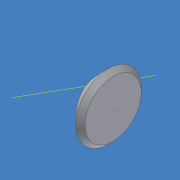
# Autodesk Inventor part: bevelgear_wheel2
Saved by Autodesk Inventor 2011 (Build 150239000, 239)
## iProperties
Created: 2005-03-17
Part Number: bevelgear_wheel2
Document SubType Name: Modeling
Designer: Miroslav Petele
Density: 1 g/cm^3
Control State: 0
Master: False
Checked Out: False
Shininess: 64.0
Angle Display Precision: 2
Document Length Units: 11269
Document Angle Units: 11279
Document Time Units: 11290
Document Mass Units: 11283
Document Length Units Precision: 3
Document Angle Units Precision: 2
Density: 0.0
Volumn: 0.0
Area: 0.0
PropertySet Name: Model Information
Author: Miroslav Petele
Autodesk Inventor part; units mm, degrees
ref_plane "YZ Plane" through (0, 0, 0) normal (1, 0, 0) x (0, 1, 0)
ref_plane "XZ Plane" through (0, 0, 0) normal (0, 1, 0) x (-1, 0, 0)
ref_plane "XY Plane" through (0, 0, 0) normal (0, 0, 1) x (1, 0, 0)
ref_plane "Work Plane1" through (0, 0, -10) normal (-0.8660254, 0.5, 0) x (-0.5, -0.8660254, 0)
sketch "Sketch1" plane through (0, 0, 0) normal (0, 0, 1) x (1, 0, 0)
  line L0 (-8.9539, 0) -> (116.4008, 0) projected
  line L1 (0, 0) -> (22.3574, 21.64) construction
  line L2 (67.2393, 58.2059) -> (103.4352, 89.5391)
  line L3 (67.2393, 58.2059) -> (68.9265, 56.4627)
  line L4 (68.9265, 56.4627) -> (68.9265, 0)
  line L5 (103.4352, 89.5391) -> (109.1987, 83.5845)
  line L6 (109.1987, 83.5845) -> (109.1987, 0)
  dimension "delta" = 44.066
  dimension "hxe" = 8.287
  dimension "hxi" = 2.426
  dimension "hfe" = 7.6
  dimension "hfi" = 4.9405
  dimension "Ri" = 88.7955
  dimension "b" = 47.8
  constraints: 12 end point, 4 perpendicular, 2 point on line
  measures "delta" angle of L0 L1
  measures "hxe" distance of L2.end L5.end
  measures "hxi" distance of L2.start L3.end
  measures "hfe" distance from line of L1 L2.end
  measures "hfi" distance from line of L1 L2.start
  measures "Ri" distance from line of L1.start L3
  measures "b" distance between parallel lines of L5 L3
revolve "Revolution1" add sketch "Sketch1" angle 360 about axis through (-10, 0, 0) along (1, 0, 0)
sketch "Sketch2" plane through (0, 0, 0) normal (0, 0, 1) x (1, 0, 0)
  line L0 (-9.7443, 0) -> (126.676, 0) projected
  line L1 (0, 0) -> (23.1863, 22.4423) construction
  line L2 (67.2393, 58.2059) -> (103.4352, 89.5391) projected
  line L3 (67.2393, 58.2059) -> (62.2661, 63.344)
  line L4 (103.4352, 89.5391) -> (95.7849, 97.443)
  line L5 (95.7849, 97.443) -> (62.2661, 63.344)
  dimension "hae" = 3.4
  dimension "hai" = 2.2102
  dimension "d10" = 44.066
  constraints: 8 end point, 1 parallel, 1 perpendicular
  measures "hae" distance from line of L1 L4.end
  measures "hai" distance from line of L1 L3.end
  measures "d10" angle of L0 L1
revolve "Revolution2" add sketch "Sketch2" angle 360 about axis through (-10, 0, 0) along (1, 0, 0)
equation "\"delta\" = MC_delta2"
equation "\"hxe\" = MC_hxe2 + MC_hae2 - MC_h2E"
equation "\"hxi\" = MC_hxi2 + MC_hai2 - MC_h2A"
equation "\"hfe\" = MC_h2E - MC_hae2"
equation "\"hfi\" = MC_h2A - MC_hai2"
equation "\"Ri\" = MC_Ri"
equation "\"b\" = MC_b"
equation "\"hae\" = MC_hae2"
equation "\"hai\" = MC_hai2"
equation "\"d10\" = delta"
equation "\"SumDelta\" = MC_deltasum"
equation "\"MC_deltasum\" = 60deg"
equation "\"MC_b\" = 47.8"
equation "\"MC_Ri\" = 88.79551"
equation "\"MC_alfa\" = 20deg"
equation "\"MC_delta1\" = 15.934197deg"
equation "\"MC_hae1\" = 6.6"
equation "\"MC_hxe1\" = 9.9"
equation "\"MC_hai1\" = 4.29041"
equation "\"MC_hxi1\" = 4.84827"
equation "\"MC_delta2\" = 44.0658deg"
equation "\"MC_hae2\" = 3.4"
equation "\"MC_hxe2\" = 15.887"
equation "\"MC_hai2\" = 2.21021"
equation "\"MC_hxi2\" = 7.36647"
equation "\"MC_Ang1A\" = 212.432024deg"
equation "\"MC_Ang1B\" = 194.292538deg"
equation "\"MC_Ang1C\" = 180deg"
equation "\"MC_Ang1D\" = 168.447967deg"
equation "\"MC_Ang1E\" = 158.917183deg"
equation "\"MC_Ang2A\" = 167.197885deg"
equation "\"MC_Ang2B\" = 174.358209deg"
equation "\"MC_Ang2C\" = 180deg"
equation "\"MC_Ang2D\" = 184.560013deg"
equation "\"MC_Ang2E\" = 188.322165deg"
equation "\"MC_h1A\" = 7.15068"
equation "\"MC_h1B\" = 8.11301"
equation "\"MC_h1C\" = 9.07534"
equation "\"MC_h1D\" = 10.03767"
equation "\"MC_h1E\" = 11"
equation "\"MC_h2A\" = 7.15068"
equation "\"MC_h2B\" = 8.11301"
equation "\"MC_h2C\" = 9.07534"
equation "\"MC_h2D\" = 10.03767"
equation "\"MC_h2E\" = 11"
equation "\"MC_Rz1A\" = 24.37731"
equation "\"MC_Rz1B\" = 27.65799"
equation "\"MC_Rz1C\" = 30.93866"
equation "\"MC_Rz1D\" = 34.21933"
equation "\"MC_Rz1E\" = 37.5"
equation "\"MC_Rz2A\" = 61.75586"
equation "\"MC_Rz2B\" = 70.0669"
equation "\"MC_Rz2C\" = 78.37793"
equation "\"MC_Rz2D\" = 86.68897"
equation "\"MC_Rz2E\" = 95"
equation "\"MC_Sa1A\" = 0.52085"
equation "\"MC_Sa1B\" = 0.59095"
equation "\"MC_Sa1C\" = 0.66104"
equation "\"MC_Sa1D\" = 0.73114"
equation "\"MC_Sa1E\" = 0.80123"
equation "\"MC_Sa2A\" = 1.22771"
equation "\"MC_Sa2B\" = 1.39293"
equation "\"MC_Sa2C\" = 1.55815"
equation "\"MC_Sa2D\" = 1.72338"
equation "\"MC_Sa2E\" = 1.8886"
equation "\"MC_tx1A\" = 5.53762"
equation "\"MC_tx1B\" = 6.28287"
equation "\"MC_tx1C\" = 7.02812"
equation "\"MC_tx1D\" = 7.77336"
equation "\"MC_tx1E\" = 8.51861"
equation "\"MC_tx2A\" = 4.02113"
equation "\"MC_tx2B\" = 4.56228"
equation "\"MC_tx2C\" = 5.10344"
equation "\"MC_tx2D\" = 5.6446"
equation "\"MC_tx2E\" = 6.18576"
equation "\"MC_bD\" = 11.95"
equation "\"MC_bC\" = 23.9"
equation "\"MC_bB\" = 35.85"
equation "\"MC_bA\" = 48.756"
equation "\"MC_mx1A\" = 2.6348"
equation "\"MC_mx1B\" = 2.98939"
equation "\"MC_mx1C\" = 3.34398"
equation "\"MC_mx1D\" = 3.69856"
equation "\"MC_mx1E\" = 4.05315"
equation "\"MC_mx2A\" = 2.50501"
equation "\"MC_mx2B\" = 2.84213"
equation "\"MC_mx2C\" = 3.17925"
equation "\"MC_mx2D\" = 3.51637"
equation "\"MC_mx2E\" = 3.8535"
body "Solid1"
